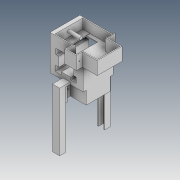
# Autodesk Inventor part: Peça16
Saved by Autodesk Inventor 2021 (Build 250183000, 183)
## iProperties
Created: 2020-10-08
Part Number: Peça16
Material: Genérico
Document SubType Name: Modeling
Designer: evert
Density: 1 g/cm^3
Appearance: Padrão
Author: evert
Autodesk Inventor part; units mm, degrees
ref_plane "YZ Plane" through (0, 0, 0) normal (1, 0, 0) x (0, 1, 0)
ref_plane "XZ Plane" through (0, 0, 0) normal (0, 1, 0) x (-1, 0, 0)
ref_plane "XY Plane" through (0, 0, 0) normal (0, 0, 1) x (1, 0, 0)
sketch "Esboço2" plane through (0, 0, 0) normal (0, 0, 1) x (1, 0, 0)
  line L0 (0, 0) -> (-5, 0)
  line L1 (-5, 0) -> (-5, -5)
  line L2 (-5, -5) -> (-2, -5)
  line L3 (-2, -5) -> (-2, -15)
  line L4 (-2, -15) -> (-5.6275, -15)
  line L5 (-5.6275, -15) -> (-5.6275, -20)
  line L6 (-5.6275, -20) -> (0, -20)
  line L7 (0, -20) -> (0, -17.5)
  line L8 (0, -17.5) -> (10, -17.5)
  line L9 (10, -17.5) -> (10, -20)
  line L10 (10, -20) -> (15, -20)
  line L11 (15, -20) -> (15, -15)
  line L12 (15, -15) -> (12.5, -15)
  line L13 (12.5, -15) -> (12.5, -5)
  line L14 (12.5, -5) -> (15, -5)
  line L15 (15, 0) -> (15, -5)
  line L16 (15, 0) -> (10, 0)
  line L17 (10, 0) -> (10, -2.5)
  line L18 (10, -2.5) -> (0, -2.5)
  line L19 (0, -2.5) -> (0, 0)
  line L20 (-2.2, -14.8) -> (-2.2, -5.2)
  line L21 (-2.2, -5.2) -> (-4.7, -5.2)
  line L22 (-2.2, -14.8) -> (-4.7, -14.8)
  line L23 (-2.2, -14.8) -> (-5.8275, -14.8)
  line L24 (-5.8275, -14.8) -> (-5.8275, -20)
  line L25 (-5.8275, -20) -> (-5.8275, -20.2)
  line L26 (-5.8275, -20.2) -> (0.2, -20.2)
  line L27 (0.2, -20.2) -> (0.2, -17.7)
  line L28 (0.2, -17.7) -> (9.8, -17.7)
  line L29 (9.8, -17.7) -> (9.8, -18.4636)
  line L30 (9.8, -18.4636) -> (9.8, -20.2)
  line L31 (9.8, -20.2) -> (15.2, -20.2)
  line L32 (15.2, -20.2) -> (15.2, -14.8)
  line L33 (15.2, -14.8) -> (12.7, -14.8)
  line L34 (12.7, -14.8) -> (12.7, -5.2)
  line L35 (12.7, -5.2) -> (15.1265, -5.2)
  line L36 (15.1265, -5.2) -> (15.2, -5.2)
  line L37 (15.2, -5.2) -> (15.2, 0)
  line L38 (-4.7, -5.2) -> (-5.2, -5.2)
  line L39 (-5.2, -5.2) -> (-5.2, 0)
  line L40 (-12.2, 0) -> (-12.2, -24.2)
  line L41 (-12.2, -24.2) -> (22.2, -24.2)
  line L42 (22.2, -24.2) -> (22.2, 0)
  line L43 (15.2, 0) -> (15.2, 0.2)
  line L44 (15.2, 0.2) -> (13.2, 0.2)
  line L45 (22.2, 0) -> (22.2, 1)
  line L46 (22.2, 1) -> (13.2, 1)
  line L47 (13.2, 1) -> (13.2, 0.2)
  line L48 (-12.2, 0) -> (-12.2, 1.2)
  line L49 (-5.2, 0) -> (-5.2, 0.2)
  line L50 (-5.2, 0.2) -> (-3.2, 0.2)
  line L51 (-3.2, 1.2) -> (-12.2, 1.2)
  line L52 (-3.2, 1.2) -> (0, 1.2)
  line L53 (0, 1.2) -> (0, 0.2)
  line L54 (0, 0.2) -> (-3.2, 0.2)
  line L55 (0.5946, -2.5) -> (0.5946, 9.5)
  line L56 (0.5946, 9.5) -> (9.5946, 9.5)
  line L57 (9.5946, 9.5) -> (9.5946, -2.5)
  line L58 (0.5946, -2.5) -> (9.5946, -2.5)
  dimension "d0" = 5
  dimension "d1" = 5
  dimension "d2" = 3
  dimension "d3" = 10
  dimension "d4" = 5
  dimension "d5" = 2.5
  dimension "d6" = 10
  dimension "d7" = 5
  dimension "d8" = 5
  dimension "d9" = 10
  dimension "d11" = 5
  dimension "d12" = 0.2
  dimension "d13" = 0.2
  dimension "d14" = 0.2
  dimension "d15" = 0.2
  dimension "d16" = 0.2
  dimension "d17" = 0.2
  dimension "d19" = 0.2
  dimension "d20" = 0.2
  dimension "d21" = 0.2
  dimension "d22" = 0.2
  dimension "d23" = 0.2
  dimension "d24" = 0.2
  dimension "d25" = 0.2
  dimension "d26" = 0.2
  dimension "d27" = 0.2
  dimension "d28" = 7
  dimension "d29" = 4
  dimension "d30" = 7
  dimension "d31" = 0.2
  dimension "d32" = 2
  dimension "d33" = 1
  dimension "d34" = 0.2
  dimension "d35" = 2
  dimension "d36" = 1
  dimension "d39" = 12
  dimension "d40" = 9
  constraints: 118 end point, 27 perpendicular, 16 point on line, 9 horizontal, 8 vertical, 3 parallel, 1 collinear
  measures "d0" distance of L0.start L0.end
  measures "d1" distance of L0.end L1.end
  measures "d2" distance of L1.end L2.end
  measures "d3" distance of L2.end L3.end
  measures "d4" distance of L4.end L5.end
  measures "d5" distance of L6.end L7.end
  measures "d6" distance of L7.end L8.end
  measures "d7" distance of L9.end L10.end
  measures "d8" distance of L10.end L11.end
  measures "d9" distance of L12.end L13.end
  measures "d11" distance of L15.start L16.end
  measures "d12" distance between parallel lines of L3 L20
  measures "d13" distance between parallel lines of L21 L2
  measures "d14" distance between parallel lines of L4 L22
  measures "d15" distance between parallel lines of L5 L24
  measures "d16" distance between parallel lines of L6 L26
  measures "d17" distance between parallel lines of L7 L27
  measures "d19" distance between parallel lines of L8 L28
  measures "d20" distance between parallel lines of L9 L29
  measures "d21" distance between parallel lines of L31 L10
  measures "d22" distance between parallel lines of L11 L32
  measures "d23" distance between parallel lines of L12 L33
  measures "d24" distance between parallel lines of L34 L13
  measures "d25" distance between parallel lines of L35 L14
  measures "d26" distance between parallel lines of L37 L15
  measures "d27" distance between parallel lines of L1 L39
  measures "d28" distance of L39.end L40.start
  measures "d29" distance from line of L41 L25.end
  measures "d30" distance from line of L42 L31.end
  measures "d31" distance of L37.end L43.end
  measures "d32" distance of L43.end L44.end
  measures "d33" distance of L42.end L45.end
  measures "d34" distance of L39.end L49.end
  measures "d35" distance of L49.end L50.end
  measures "d36" distance between parallel lines of L50 L51
  measures "d39" distance of L55.start L55.end
  measures "d40" distance of L55.end L56.end
extrude "Extrusão1" add sketch "Esboço2" along normal blind 30 contours L22 L23 L24 L25 L26 L27 L28 L29 L30 L31 L32 L33 L34 L35 L36 L37 L43 L44 L47 L46 L45 L42 L41 L40 L48 L51 L52 L53 L54 L50 L49 L39 L38 L21 L20
sketch "Esboço4" plane through (-12.2, -24.2, 0) normal (-1, 0, 0) x (0, 0, 1)
  circle A0 centre (30, 27.7) radius 6 projected
  line L0 (30, 27.7) -> (0, 27.7)
  line L1 (15, 27.7) -> (15, 25.4)
  line L2 (0, 25.4) -> (30, 25.4) projected
  line L3 (0, 27.7) -> (30, 27.7)
  line L4 (30, 27.7) -> (30, 25.4)
  line L5 (30, 25.4) -> (0, 25.4)
  line L6 (0, 25.4) -> (0, 27.7)
  point P0 (0, 24.2)
  constraints: 12 end point, 2 horizontal, 2 midpoint, 2 parallel, 1 perpendicular
extrude "Extrusão2" add sketch "Esboço4" against normal blind 5 contours L0 L4 L2 A0 | A0 L2 L1 L0 | L1 L2 L6 L0 picked at (28.1528, 26.1667)
sketch "Esboço5" plane through (-7.2, -24.2, 0) normal (1, 0, 0) x (0, 0, -1)
  line L0 (-30, 27.7) -> (0, 27.7) projected
  line L1 (0, 27.7) -> (-15, 27.7)
  circle A0 centre (-15, 27.7) radius 1.5
  point P0 (0, 24.2)
  dimension "d48" = 3
  constraints: 2 end point, 1 centre point, 1 coincident, 1 midpoint
  measures "d48" diameter of A0
extrude "Extrusão3" add sketch "Esboço5" along normal blind 12.2
sketch "Esboço6" plane through (-7.2, -24.2, 0) normal (-1, 0, 0) x (0, 0, 1)
  line L0 (13.5, 27.7) -> (16.5, 27.7) projected
  circle A0 centre (15, 27.7) radius 1.5
  point P0 (0, 24.2)
  constraints: 1 centre point, 1 midpoint
extrude "Extrusão4" add sketch "Esboço6" along normal blind 5 contours A0 L0 picked at (15.4855, 27.8197)
sketch "Esboço7" plane through (-12.2, -24.2, 0) normal (-1, 0, 0) x (0, 0, 1)
  circle A0 centre (30, 27.7) radius 6 projected
  line L0 (13.5, 27.7) -> (0, 27.7) projected
  line L1 (30, 33.7) -> (0, 33.7)
  line L2 (0, 33.7) -> (0, 27.7)
  line L3 (0, 27.7) -> (30, 27.7)
  line L4 (30, 27.7) -> (30, 33.7)
  point P0 (0, 24.2)
  constraints: 8 end point, 2 parallel, 1 horizontal, 1 perpendicular, 1 vertical alignment, 1 other
extrude "Extrusão5" add sketch "Esboço7" against normal blind 5 contours L4 L3 A0 | A0 L3 L0 L2 L1 picked at (26.0501, 28.145)
sketch "Esboço8" plane through (-12.2, -24.2, 0) normal (-1, 0, 0) x (0, 0, 1)
  line L0 (30, 33.7) -> (0, 33.7) projected
  line L1 (0, 33.7) -> (0, 35.2)
  line L2 (0, 35.2) -> (30, 35.2)
  line L3 (30, 35.2) -> (30, 33.7)
  line L4 (30, 33.7) -> (0, 33.7)
  line L5 (30, 33.7) -> (30, 25.4) projected
  point P0 (0, 24.2)
  dimension "d55" = 1.5
  constraints: 8 end point, 3 perpendicular, 1 vertical
  measures "d55" distance of L0.end L1.end
extrude "Extrusão6" add sketch "Esboço8" against normal blind 5
sketch "Esboço10" plane through (13.2, 1, 0) normal (0, 1, 0) x (1, 0, 0)
  line L0 (-8.2, -16.5) -> (-8.2, -13.5) projected
  line L1 (-8.2, -15) -> (-8.2, -21.5)
  line L2 (-8.2, -15) -> (-8.2, -8.5)
  line L3 (0, 0) -> (0, -30) projected
  line L4 (0, 0) -> (-13.2, 0)
  line L5 (-3.4, 0) -> (-13, 0) projected
  line L6 (-13.2, 0) -> (-13.2, -8.5)
  line L7 (-13, 0) -> (-13, -30) projected
  line L8 (-13.2, -8.5) -> (0, -8.5)
  line L9 (0, -8.5) -> (0, 0)
  line L10 (2, -30) -> (-3.4, -30) projected
  line L11 (0, -30) -> (0, -21.5)
  line L12 (0, -21.5) -> (-13.2, -21.5)
  line L13 (-13.2, 0) -> (-13.2, -30) projected
  line L14 (-13.2, -21.5) -> (-13.2, -30)
  line L15 (-13.2, -30) -> (0, -30)
  dimension "d58" = 6.5
  dimension "d59" = 6.5
  constraints: 20 end point, 5 perpendicular, 5 point on line, 2 collinear, 1 midpoint, 1 parallel
  measures "d58" distance of L1.start L1.end
  measures "d59" distance of L1.start L2.end
extrude "Extrusão7" add sketch "Esboço10" against normal blind 0.8 contours L12 L3 L10 L15 L7 | L7 L15 L13 L12 | L8 L7 L4 L3 | L8 L6 L4 L7
sketch "Esboço15" plane through (22.2, -24.2, 0) normal (1, 0, 0) x (0, 0, -1)
  line L0 (-30, 25.2) -> (-21.5, 25.2) projected
  line L1 (-30, 25.2) -> (0, 25.2)
  line L2 (0, 25.2) -> (0, 24.2)
  line L3 (0, 24.2) -> (-30, 24.2)
  line L4 (-30, 24.2) -> (-30, 25.2)
  constraints: 8 end point, 2 parallel, 1 horizontal, 1 perpendicular
extrude "Extrusão10" add sketch "Esboço15" along normal blind 3
sketch "Esboço16" plane through (0, 1, 8.5) normal (0, 1, 0) x (1, 0, 0)
  line L0 (22.2, -21.5) -> (25.2, -21.5) projected
  line L1 (25.2, 8.5) -> (23.7, 8.5)
  line L2 (23.7, -21.5) -> (25.2, -21.5)
  line L3 (0, -21.5) -> (25.2, -21.5) projected
  line L4 (-12.2, -21.5) -> (-12.2, 8.5) projected
  line L5 (25.2, -21.5) -> (-12.2, -21.5)
  line L6 (-12.2, -21.5) -> (-12.2, -20.5)
  line L7 (-12.2, -20.5) -> (25.2, -20.5)
  line L8 (25.2, -20.5) -> (25.2, -21.5)
  line L9 (0, 8.5) -> (25.2, 8.5) projected
  line L10 (25.2, 8.5) -> (-12.2, 8.5)
  line L11 (-12.2, 8.5) -> (-12.2, 7.5)
  line L12 (-12.2, 7.5) -> (25.2, 7.5)
  line L13 (25.2, 7.5) -> (25.2, 8.5)
  line L14 (25.2, 8.5) -> (24.2, 8.5)
  line L15 (24.2, 8.5) -> (24.2, -21.5)
  line L16 (24.2, -21.5) -> (25.2, -21.5)
  line L17 (25.2, -21.5) -> (25.2, 8.5)
  point P0 (24.2, 7.5)
  point P1 (24.2, -20.5)
  dimension "d70" = 1
  dimension "d71" = 1
  dimension "d73" = 1
  constraints: 28 end point, 7 parallel, 4 horizontal, 3 perpendicular, 3 point on line, 1 midpoint
  measures "d70" distance between parallel lines of L9 L12
  measures "d71" distance between parallel lines of L7 L3
  measures "d73" distance of L16.end L15.end
extrude "Extrusão11" add sketch "Esboço16" along normal blind 10 contours L3 L5 L4 L7 L15 L0 | L15 L7 L8 L0 | L15 L12 L17 L7 | L15 L1 L13 L12 | L12 L4 L10 L9 L1 L15
sketch "Esboço18" plane through (0, 0, 30) normal (0, 0, 1) x (1, 0, 0)
  line L0 (-12.2, 11) -> (-12.2, -24.2) projected
  line L1 (-12.2, -24.2) -> (22.2, -24.2) projected
  line L2 (-12.2, 11) -> (-11.2, 11)
  line L3 (-11.2, 11) -> (-11.2, -24.2)
  line L4 (-11.2, -24.2) -> (-12.2, -24.2)
  line L5 (-12.2, -24.2) -> (-12.2, 11)
  point P0 (0, 0)
  dimension "d76" = 1
  constraints: 8 end point, 2 parallel, 1 horizontal, 1 perpendicular, 1 point on line
  measures "d76" distance of L3.end L4.end
extrude "Extrusão12" cut sketch "Esboço18" against normal through all
sketch "Esboço20" plane through (0, 1, 8.5) normal (0, 1, 0) x (1, 0, 0)
  line L0 (0, 7.5) -> (0, -20.5) projected
  line L1 (12.7, 8.5) -> (12.7, -21.5) projected
  line L2 (0, 0) -> (12.7, 0)
  line L3 (12.7, 0) -> (12.7, 1)
  line L4 (12.7, 1) -> (0, 1)
  line L5 (0, 1) -> (0, 0)
  line L6 (0, 0) -> (13.2, 0) projected
  line L7 (12.7, 1) -> (13.2, 1)
  line L8 (13.2, 1) -> (13.2, 0)
  line L9 (13.2, 0) -> (12.7, 0)
  line L10 (12.7, 0) -> (12.7, 1)
  line L11 (13.2, 0) -> (13.2, -13) projected
  line L12 (0, -20.5) -> (0, -13) projected
  line L13 (13.2, -13) -> (0, -13)
  line L14 (0, -13) -> (0, -14)
  line L15 (0, -14) -> (13.2, -14)
  line L16 (13.2, -14) -> (13.2, -13)
  point P0 (0, 8.5)
  point P1 (0, -14)
  point P2 (0, -13)
  point P3 (0, 1)
  dimension "d79" = 1
  dimension "d80" = 1
  constraints: 24 end point, 6 parallel, 3 horizontal, 3 perpendicular, 3 point on line
  measures "d79" distance between parallel lines of L4 L2
  measures "d80" distance between parallel lines of L15 L13
extrude "Extrusão13" cut sketch "Esboço20" against normal blind 1 contours L4 L1 L2 L0 | L7 L8 L6 L1 | L13 L1 L15 L0 | L13 L16 L15 L1
sketch "Esboço38" plane through (22.2, -24.2, 0) normal (0, -1, 0) x (1, 0, 0)
  line L0 (-33.4, 0) -> (-33.4, 30) projected
  line L1 (0, 0) -> (-33.4, 0)
  line L2 (-33.4, 0) -> (-33.4, 30)
  line L3 (-33.4, 30) -> (0, 30)
  line L4 (0, 30) -> (0, 0)
  line L5 (0, 0) -> (0, 3.5)
  line L6 (-33.4, 30) -> (0, 30) projected
  line L7 (0, 30) -> (0, 26.5)
  line L8 (0, 26.5) -> (0, 3.5)
  line L9 (0, 3.5) -> (-16.5, 3.5)
  line L10 (0, 26.5) -> (-16.5, 26.5)
  line L11 (-16.5, 3.5) -> (-16.5, 26.5)
  line L12 (0, 3.5) -> (0, 3)
  line L13 (0, 0) -> (0, 30) projected
  line L14 (0, 3) -> (-17, 3)
  line L15 (-17, 3) -> (-17, 3.5)
  line L16 (-17, 3.5) -> (-16.5, 3.5)
  line L17 (0, 26.5) -> (0, 27)
  line L18 (0, 27) -> (-17, 27)
  line L19 (-17, 27) -> (-17, 26.5)
  line L20 (-17, 26.5) -> (-16.5, 26.5)
  line L21 (0, 3.5) -> (-0.5, 3.5)
  line L22 (-0.5, 3.5) -> (-0.5, 26.5)
  point P0 (-22.2, 0)
  point P1 (0, 27)
  dimension "d128" = 3.5
  dimension "d129" = 3.5
  dimension "d131" = 16.5
  dimension "d132" = 16.5
  dimension "d133" = 0.5
  dimension "d134" = 17
  dimension "d135" = 0.5
  constraints: 40 end point, 8 point on line, 6 perpendicular, 3 horizontal, 2 parallel, 1 vertical
  measures "d128" distance of L1.start L5.end
  measures "d129" distance of L6.end L7.end
  measures "d131" distance of L5.end L9.end
  measures "d132" distance of L7.end L10.end
  measures "d133" distance of L5.end L12.end
  measures "d134" distance of L12.end L14.end
  measures "d135" distance of L7.end L17.end
extrude "Extrusão25" add sketch "Esboço38" along normal blind 12 contours L14 L15 L16 L9 L4 | L4 L10 L20 L19 L18 | L9 L22 L10 L4
sketch "Esboço39" plane through (22.2, -36.2, 0) normal (0, -1, 0) x (1, 0, 0)
  line L0 (-17, 3) -> (0, 3) projected
  line L1 (0, 27) -> (-17, 27) projected
  line L2 (0, 3) -> (-17, 3)
  line L3 (-17, 3) -> (-17, 27)
  line L4 (-17, 27) -> (0, 27)
  line L5 (0, 27) -> (0, 3)
  point P0 (-22.2, 0)
  point P1 (-17, 3)
  constraints: 8 end point, 2 parallel, 1 horizontal, 1 perpendicular
extrude "Extrusão26" add sketch "Esboço39" along normal blind 1
sketch "Esboço40" plane through (5.2, -24.2, 27) normal (0, 0, 1) x (1, 0, 0)
  line L0 (0, -13) -> (17, -13) projected
  line L1 (0, 0) -> (16.5, 0) projected
  line L2 (0, -13) -> (1, -13)
  line L3 (1, -13) -> (1, 0)
  line L4 (1, 0) -> (0, 0)
  line L5 (0, 0) -> (0, -13)
  point P0 (-5.2, 24.2)
  point P1 (1, -13)
  dimension "d140" = 1
  constraints: 8 end point, 2 parallel, 1 horizontal, 1 perpendicular, 1 point on line
  measures "d140" distance of L4.end L3.end
extrude "Extrusão27" add sketch "Esboço40" along normal blind 5
sketch "Esboço41" plane through (22.2, -24.2, 3) normal (0, 0, -1) x (-1, 0, 0)
  line L0 (17, 0) -> (17, -13) projected
  line L1 (16, 0) -> (16, -13) projected
  line L2 (17, 0) -> (16, 0)
  line L3 (16, 0) -> (16, -13)
  line L4 (16, -13) -> (17, -13)
  line L5 (17, -13) -> (17, 0)
  point P0 (22.2, 24.2)
  constraints: 8 end point, 2 parallel, 1 horizontal, 1 perpendicular
extrude "Extrusão28" add sketch "Esboço41" along normal blind 5
sketch "Esboço42" plane through (5.2, -36.2, 3.5) normal (-1, 0, 0) x (0, 0, 1)
  line L0 (-5.5, -1) -> (-5.5, 12) projected
  line L1 (-5.5, 12) -> (-5.5, 6.1)
  line L2 (-5.5, 6.1) -> (0, 6.1)
  line L3 (0, 12) -> (0, 0) projected
  line L4 (0, 6.1) -> (28.5, 6.1)
  line L5 (28.5, -1) -> (28.5, 12) projected
  line L6 (-5.5, 6.1) -> (-2.75, 6.1)
  circle A0 centre (-2.75, 6.1) radius 0.5
  line L7 (28.5, 6.1) -> (25.75, 6.1)
  circle A1 centre (25.75, 6.1) radius 0.5
  point P0 (-3.5, 36.2)
  dimension "d145" = 5.9
  dimension "d146" = 1
  dimension "d147" = 2.75
  dimension "d148" = 1
  constraints: 10 end point, 5 point on line, 2 centre point, 2 coincident, 1 horizontal, 1 midpoint
  measures "d145" distance of L0.end L1.end
  measures "d146" diameter of A0
  measures "d147" distance of L4.end L7.end
  measures "d148" diameter of A1
extrude "Extrusão29" cut sketch "Esboço42" against normal blind 5
sketch "Esboço46" plane through (22.2, -37.2, 0) normal (0, -1, 0) x (1, 0, 0)
  line L0 (-17, -2) -> (-17, 32) projected
  line L1 (-17, 26.9875) -> (-19, 26.9875)
  line L2 (-22.2, 29) -> (-22.2, 22.5) projected
  line L3 (-19, 26.9875) -> (-19, 3.5)
  line L4 (-17, 0) -> (-17, 3.5) projected
  line L5 (-19, 3.5) -> (-17, 3.5)
  point P0 (-22.2, 0)
  dimension "d152" = 2
  constraints: 6 end point, 3 perpendicular, 1 point on line
  measures "d152" distance of L1.start L1.end
extrude "Extrusão30" add sketch "Esboço46" against normal blind 1
sketch "Esboço47" plane through (22.2, -37.2, 0) normal (0, -1, 0) x (1, 0, 0)
  line L0 (-16.7452, 15.2437) -> (-16.7452, 11.1125)
  line L1 (-16.7452, 11.1125) -> (-16.7452, 15.2437)
  line L2 (-16.7452, 19.05) -> (-16.7452, 15.2437)
  line L3 (-16.7452, 15.2437) -> (-16.7452, 17.2437)
  line L4 (-16.7452, 17.2437) -> (-17.2452, 17.2437)
  line L5 (-17.2452, 17.2437) -> (-16.7452, 17.2437)
  line L6 (-16.7452, 17.2437) -> (-16.2452, 17.2437)
  line L7 (-16.2452, 17.2437) -> (-16.2452, 16.2437)
  line L8 (-29.4, 16.5) -> (-17.2, 16.5) projected
  line L9 (-16.2452, 16.2437) -> (-17.2452, 16.2437)
  line L10 (-17.2452, 16.2437) -> (-17.2452, 17.2437)
  line L11 (-16.7452, 15.2437) -> (-16.7452, 13.2437)
  line L12 (-16.7452, 13.2437) -> (-17.2452, 13.2437)
  line L13 (-17.2452, 13.2437) -> (-16.7452, 13.2437)
  line L14 (-16.2452, 13.2437) -> (-16.7452, 13.2437)
  line L15 (-29.4, 13.5) -> (-17.2, 13.5) projected
  line L16 (-16.2452, 13.2437) -> (-16.2452, 14.2437)
  line L17 (-16.2452, 14.2437) -> (-17.2452, 14.2437)
  line L18 (-17.2452, 14.2437) -> (-17.2452, 13.2437)
  point P0 (-22.2, 0)
  dimension "d155" = 2
  dimension "d156" = 0.5
  dimension "d157" = 0.5
  dimension "d158" = 2
  constraints: 34 end point, 9 point on line, 7 perpendicular, 4 collinear, 1 parallel, 1 vertical
  measures "d155" distance of L0.start L3.end
  measures "d156" distance of L3.end L4.end
  measures "d157" distance of L3.end L6.end
  measures "d158" distance of L0.start L11.end
extrude "Extrusão31" add sketch "Esboço47" along normal blind 3
sketch "Esboço48" plane through (5.9548, -37.2, 16.2437) normal (0, 0, -1) x (-1, 0, 0)
  line L0 (0, -3) -> (1, -3) projected
  circle A0 centre (0.5, -3) radius 0.5
  point P0 (5.9548, 37.2)
  dimension "d161" = 1
  constraints: 1 centre point, 1 midpoint
  measures "d161" diameter of A0
extrude "Extrusão32" add sketch "Esboço48" along normal blind 3 and the other way blind 1
sketch "Esboço53" plane through (0, 1, 29) normal (0, 1, 0) x (1, 0, 0)
  line L0 (13.2, 21.5) -> (13.2, 6.5) projected
  line L1 (13.2, 21.5) -> (11.2, 21.5)
  line L2 (13.2, 21.5) -> (0, 21.5) projected
  line L3 (11.2, 21.5) -> (11.2, 6.5)
  line L4 (0, 6.5) -> (13.2, 6.5) projected
  line L5 (13.2, 6.5) -> (11.2, 6.5)
  line L6 (13.2, 6.5) -> (13.2, 21.5)
  point P0 (0, 29)
  dimension "d169" = 2
  constraints: 8 end point, 3 perpendicular, 2 point on line
  measures "d169" distance of L0.start L1.end
extrude "Extrusão34" add sketch "Esboço53" against normal blind 0.8
sketch "Esboço54" plane through (25.2, 11, 30) normal (0, 1, 0) x (1, 0, 0)
  line L0 (-1, 1) -> (-1, 29) projected
  line L1 (-1, 1) -> (0, 1)
  line L2 (0, 1) -> (0, 29)
  line L3 (0, 0) -> (0, 30) projected
  line L4 (-1, 29) -> (-25.2, 29) projected
  line L5 (-1, 29) -> (0, 29)
  line L6 (-25.2, 1) -> (-1, 1) projected
  line L7 (-1, 29) -> (-1, 1)
  point P0 (-25.2, 30)
  constraints: 8 end point, 1 collinear, 1 horizontal, 1 perpendicular, 1 point on line
extrude "Extrusão35" cut sketch "Esboço54" against normal blind 10
sketch "Esboço57" plane through (-7.2, -24.2, 0) normal (1, 0, 0) x (0, 0, -1)
  line L0 (-1, 25.4) -> (-1, 35.2) projected
  circle A0 centre (-15, 27.7) radius 1.5 projected
  circle A1 centre (-15, 30.7) radius 1.5
  line L1 (-15, 27.7) -> (-15, 30.7)
  point P0 (0, 24.2)
  dimension "d175" = 3
  constraints: 2 end point, 1 centre point, 1 vertical
  measures "d175" diameter of A1
extrude "Extrusão36" add sketch "Esboço57" along normal blind 12.2 contours A1
sketch "Esboço58" plane through (5, 3.5, 15) normal (1, 0, 0) x (0, 0, -1)
  circle A0 centre (0, 0) radius 1.5 projected
  circle A1 centre (0, 0) radius 1.5
  point P0 (15, -3.5)
  point P1 (0, 1.5)
  constraints: 1 centre point, 1 coincident, 1 vertical alignment
extrude "Extrusão37" cut sketch "Esboço58" against normal blind 12.2
sketch "Esboço59" plane through (0, 1, 29) normal (0, 1, 0) x (1, 0, 0)
  line L0 (0, 21.5) -> (11.2, 21.5) projected
  line L1 (0, 21.5) -> (11.2, 21.5)
  line L2 (11.2, 21.5) -> (11.2, 24.5)
  line L3 (11.2, 24.5) -> (0, 24.5)
  line L4 (0, 24.5) -> (0, 21.5)
  line L5 (11.2, 6.5) -> (11.2, 21.5) projected
  line L6 (0, 0) -> (0, 6.5) projected
  line L7 (11.2, 6.5) -> (0, 6.5)
  line L8 (0, 6.5) -> (0, 3.25)
  line L9 (11.2, 6.5) -> (11.2, 3.5)
  line L10 (11.2, 3.5) -> (0, 3.5)
  point P0 (0, 29)
  point P1 (11.2, 21.5)
  point P2 (0, 3.5)
  dimension "d180" = 3
  dimension "d181" = 3
  constraints: 16 end point, 3 perpendicular, 2 horizontal, 2 parallel, 1 midpoint, 1 point on line, 1 vertical
  measures "d180" distance of L1.end L2.end
  measures "d181" distance of L5.start L9.end
extrude "Extrusão38" cut sketch "Esboço59" against normal blind 1
sketch "Esboço60" plane through (0, 1, 29) normal (0, 1, 0) x (1, 0, 0)
  line L0 (25.2, -1) -> (25.2, 29) projected
  line L1 (25.2, 29) -> (25.2, 19.54)
  line L2 (25.2, 19.54) -> (36.7, 19.54)
  line L3 (36.7, 19.54) -> (36.7, 0)
  line L4 (36.7, 0) -> (25.4, 0)
  line L5 (25.4, 0) -> (36.7, 0)
  line L6 (36.7, 19.54) -> (36.7, -2.46)
  line L7 (36.7, -2.46) -> (25.2, -2.46)
  line L8 (25.2, -2.46) -> (25.2, 19.54)
  point P0 (0, 29)
  dimension "d184" = 9.46
  dimension "d185" = 11.5
  dimension "d186" = 22
  dimension "d187" = 11.5
  constraints: 16 end point, 2 point on line, 1 horizontal, 1 parallel, 1 perpendicular, 1 vertical
  measures "d184" distance of L0.end L1.end
  measures "d185" distance of L1.end L2.end
  measures "d186" distance of L2.end L6.end
  measures "d187" distance of L6.end L7.end
extrude "Extrusão39" add sketch "Esboço60" against normal blind 1
sketch "Esboço62" plane through (-7.2, 11, 29) normal (0, 1, 0) x (1, 0, 0)
  line L0 (19.9, 29) -> (19.9, -1) projected
  line L1 (19.9, -1) -> (19.9, -4.091)
  line L2 (22.4, -1) -> (19.9, -1) projected
  line L3 (19.9, 0) -> (19.9, -1)
  line L4 (-4, -1) -> (32.4, -1) projected
  line L5 (19.9, -1) -> (32.4, -1)
  line L6 (7.2, 0) -> (32.4, 0) projected
  line L7 (32.4, -1) -> (32.4, 0)
  line L8 (32.4, 0) -> (19.9, 0)
  line L9 (32.4, 28) -> (32.4, 0) projected
  line L10 (32.4, 28) -> (32.4, 29)
  line L11 (29.4, 29) -> (32.4, 29) projected
  line L12 (32.4, 29) -> (29.4, 29)
  line L13 (29.4, 29) -> (29.4, 28)
  line L14 (32.4, 28) -> (7.2, 28) projected
  point P0 (7.2, 29)
  point P1 (32.4, 20.04)
  constraints: 16 end point, 3 collinear, 2 perpendicular, 2 point on line, 2 vertical
extrude "Extrusão41" cut sketch "Esboço62" against normal blind 10 contours L6 L7 L4 L2 L0 | L13 L11 L10 L14
sketch "Esboço64" plane through (0, 1, 4.5) normal (0, 1, 0) x (1, 0, 0)
  line L0 (22.3, -4.46) -> (25.2, -4.46) projected
  line L1 (22.2, 4.5) -> (25.2, 4.5) projected
  line L2 (22.3, -4.46) -> (25.2, -4.46)
  line L3 (25.2, -4.46) -> (25.2, 4.5)
  line L4 (25.2, 4.5) -> (22.3, 4.5)
  line L5 (22.3, 4.5) -> (22.3, -4.46)
  point P0 (0, 4.5)
  constraints: 8 end point, 2 parallel, 1 horizontal, 1 perpendicular
extrude "Extrusão43" cut sketch "Esboço64" against normal blind 12
sketch "Esboço65" plane through (0, 1, 4.5) normal (0, 1, 0) x (1, 0, 0)
  line L0 (37.2, -4.46) -> (37.2, -27.46)
  line L1 (25.2, -27.46) -> (37.2, -27.46) projected
  line L2 (37.2, -27.46) -> (22.3, -27.46)
  line L3 (22.3, -31.96) -> (22.3, -27.46) projected
  line L4 (22.3, -27.46) -> (22.3, -31.96)
  line L5 (12.7, -25.5) -> (12.7, -24.5) projected
  line L6 (12.7, -31.96) -> (12.7, -25.5)
  line L7 (12.7, -25.5) -> (25.2, -25.5)
  line L8 (15.2, 4.5) -> (15.2, -25.5) projected
  line L9 (25.2, -26.96) -> (25.2, -25.5) projected
  line L10 (25.2, -25.5) -> (25.2, -26.96)
  line L11 (36.7, -26.96) -> (25.2, -26.96) projected
  line L12 (25.2, -26.96) -> (36.7, -26.96)
  line L13 (36.7, -4.96) -> (36.7, -26.96) projected
  line L14 (36.7, -26.96) -> (36.7, -4.96)
  line L15 (36.7, -4.96) -> (21.8, -4.96)
  line L16 (25.2, -4.96) -> (36.7, -4.96) projected
  line L17 (21.8, -4.96) -> (21.8, 0.04) projected
  line L18 (21.8, -4.96) -> (21.8, 0.04)
  line L19 (21.8, 0.04) -> (22.3, 0.04)
  line L20 (22.3, 4.5) -> (22.3, -4.46) projected
  line L21 (22.3, 0.04) -> (22.3, -4.46)
  line L22 (22.3, -4.46) -> (37.2, -4.46)
  line L23 (12.7, 4.5) -> (12.7, -25.5) projected
  line L24 (12.7, -25.5) -> (12.7, -31.96)
  line L25 (12.7, -31.96) -> (12.7, -32.46)
  line L26 (12.7, -32.46) -> (22.3, -32.46)
  line L27 (22.3, -32.46) -> (22.3, -31.96)
  point P0 (0, 4.5)
  dimension "d210" = 0.5
  constraints: 34 end point, 7 collinear, 7 perpendicular, 2 point on line
  measures "d210" distance of L6.start L25.end
extrude "Extrusão44" add sketch "Esboço65" against normal blind 1
sketch "Esboço67" plane through (0, 1, 4.5) normal (0, 1, 0) x (1, 0, 0)
  line L0 (22.2, 3.5) -> (0, 3.5) projected
  line L1 (21.8, 3.5) -> (22.3, 3.5)
  line L2 (22.3, 4.5) -> (22.3, -4.46) projected
  line L3 (22.2, 4.5) -> (22.3, 4.5) projected
  line L4 (22.3, 4.5) -> (24.3, 4.5)
  line L5 (24.3, 4.5) -> (24.3, -2.46)
  line L6 (24.3, -2.46) -> (39.2, -2.46)
  line L7 (37.2, -4.46) -> (22.3, -4.46) projected
  line L8 (39.2, -2.46) -> (39.2, -29.46)
  line L9 (39.2, -29.46) -> (23.2371, -29.46)
  line L10 (23.2371, -29.46) -> (23.2371, -34.46)
  line L11 (23.2371, -34.46) -> (12.7, -34.46)
  line L12 (12.7, -32.46) -> (12.7, -25.5) projected
  line L13 (12.7, -34.46) -> (12.7, -32.46)
  line L14 (25.2, -27.46) -> (37.2, -27.46) projected
  line L15 (37.2, -27.46) -> (37.2, -4.46) projected
  line L16 (12.7, -32.46) -> (22.3, -32.46) projected
  line L17 (22.3, 4.5) -> (22.3, -4.46)
  line L18 (22.3, -4.46) -> (37.2, -4.46) projected
  line L19 (22.3, -4.46) -> (37.2, -4.46)
  line L20 (37.2, -4.46) -> (37.2, -27.46) projected
  line L21 (37.2, -4.46) -> (37.2, -27.46)
  line L22 (22.3, -31.96) -> (22.3, -27.46) projected
  line L23 (37.2, -27.46) -> (22.3, -27.46)
  line L24 (22.3, -32.46) -> (22.3, -27.46)
  line L25 (22.3, -32.46) -> (12.7, -32.46)
  point P0 (0, 4.5)
  dimension "d218" = 2
  dimension "d219" = 2
  dimension "d220" = 2
  dimension "d221" = 2
  dimension "d222" = 2
  constraints: 30 end point, 7 perpendicular, 3 collinear, 3 horizontal, 1 point on line, 1 vertical
  measures "d218" distance of L2.start L4.end
  measures "d219" distance between parallel lines of L6 L7
  measures "d220" distance between parallel lines of L14 L9
  measures "d221" distance between parallel lines of L8 L15
  measures "d222" distance between parallel lines of L11 L16
extrude "Extrusão46" add sketch "Esboço67" against normal blind 1
sketch "Esboço68" plane through (0, 1, 4.5) normal (0, 1, 0) x (1, 0, 0)
  line L0 (24.3, 4.5) -> (22.2, 4.5) projected
  line L1 (22.2, 4.5) -> (24.3, 4.5)
  line L2 (24.3, -2.46) -> (24.3, 4.5) projected
  line L3 (24.3, 4.5) -> (24.3, -2.46)
  line L4 (24.3, -2.46) -> (39.2, -2.46) projected
  line L5 (24.3, -2.46) -> (39.2, -2.46)
  line L6 (39.2, -2.46) -> (39.2, -29.46) projected
  line L7 (39.2, -2.46) -> (39.2, -29.46)
  line L8 (39.2, -29.46) -> (23.2371, -29.46) projected
  line L9 (39.2, -29.46) -> (23.2371, -29.46)
  line L10 (23.2371, -29.46) -> (23.2371, -34.46) projected
  line L11 (23.2371, -29.46) -> (23.2371, -34.46)
  line L12 (23.2371, -34.46) -> (12.7, -34.46) projected
  line L13 (23.2371, -34.46) -> (12.7, -34.46)
  line L14 (12.7, -25.5) -> (12.7, -24.5) projected
  line L15 (12.7, -34.46) -> (12.7, -24.5)
  line L16 (12.7, -24.5) -> (13.7, -24.5)
  line L17 (13.7, -24.5) -> (13.7, -33.46)
  line L18 (13.7, -33.46) -> (22.2371, -33.46)
  line L19 (22.2371, -33.46) -> (22.2371, -28.46)
  line L20 (22.2371, -28.46) -> (38.2, -28.46)
  line L21 (38.2, -28.46) -> (38.2, -3.46)
  line L22 (38.2, -3.46) -> (23.3, -3.46)
  line L23 (23.3, -3.46) -> (23.3, 3.5)
  line L24 (-7.2, 3.5) -> (22.2, 3.5) projected
  line L25 (22.2, 3.5) -> (23.3, 3.5)
  line L26 (22.2, 3.5) -> (22.2, 4.5) projected
  line L27 (22.2, 3.5) -> (22.2, 4.5)
  line L28 (22.2371, -28.46) -> (22.2371, -27.46)
  line L29 (23.2371, -29.46) -> (39.2, -29.46) projected
  line L30 (23.2371, -29.46) -> (23.2371, -28.46)
  line L31 (22.2371, -27.46) -> (38.2, -27.46)
  line L32 (23.2371, -28.46) -> (38.2, -28.46)
  line L33 (38.2, -28.46) -> (38.2, -29.46)
  line L34 (38.2, -28.46) -> (39.2, -28.46)
  line L35 (23.3, -3.46) -> (23.3, -4.46)
  line L36 (23.3, -4.46) -> (38.2, -4.46)
  line L37 (38.2, -4.46) -> (38.2, -2.46)
  line L38 (24.3, -2.46) -> (24.3, -4.46)
  line L39 (38.2, -3.46) -> (39.2, -3.46)
  line L40 (23.3, -4.46) -> (23.3, -34.46)
  line L41 (23.3, -34.46) -> (24.3, -34.46)
  line L42 (24.3, -34.46) -> (24.3, -3.46)
  line L43 (23.3, -27.46) -> (24.3, -27.46)
  line L44 (22.2371, -33.46) -> (24.3, -33.46)
  line L45 (24.3, -33.46) -> (24.3, -34.46)
  line L46 (22.2371, -34.46) -> (22.2371, -33.46)
  line L47 (22.2371, -34.46) -> (24.3, -34.46)
  point P0 (0, 4.5)
  point P1 (24.3, -3.46)
  point P2 (24.3, -28.46)
  point P3 (23.3, -33.46)
  dimension "d225" = 1
  dimension "d226" = 1
  dimension "d227" = 1
  dimension "d228" = 1
  dimension "d229" = 1
  dimension "d230" = 1
  dimension "d231" = 1
  dimension "d236" = 1
  dimension "d237" = 1
  constraints: 74 end point, 16 point on line, 15 perpendicular, 10 collinear, 5 vertical, 2 horizontal, 1 midpoint, 1 parallel
  measures "d225" distance of L14.end L16.end
  measures "d226" distance between parallel lines of L18 L12
  measures "d227" distance between parallel lines of L10 L19
  measures "d228" distance between parallel lines of L20 L8
  measures "d229" distance between parallel lines of L2 L23
  measures "d230" distance between parallel lines of L4 L22
  measures "d231" distance between parallel lines of L6 L21
  measures "d236" distance of L19.end L28.end
  measures "d237" distance of L22.end L35.end
extrude "Extrusão47" add sketch "Esboço68" along normal blind 12 contours L2 L38 L22 L23 L25 L26 L0 | L38 L36 L35 L22 | L22 L21 L36 L38 | L39 L6 L34 L21 | L42 L20 L40 L31 | L31 L21 L20 L42 | L42 L8 L40 L20 | L42 L44 L40 L8 | L42 L41 L40 L44 | L46 L12 L15 L14 L16 L17 L18 | L44 L10 L12 L46 | L40 L47 L10 L44
fillet "Arredondamento5" radius 2 1 edges at (13.2, 13, 29)
fillet "Arredondamento6" radius 2 1 edges at (22.2, 13, 0.5)
sketch "Esboço69" plane through (0, 1, 4.5) normal (0, 1, 0) x (1, 0, 0)
  line L0 (39.2, -2.46) -> (39.2, -29.46) projected
  line L1 (39.2, -3.46) -> (24.3, -3.46) projected
  line L2 (39.2, -2.46) -> (24.3, -2.46)
  line L3 (24.3, -2.46) -> (24.3, -3.46)
  line L4 (24.3, -3.46) -> (39.2, -3.46)
  line L5 (39.2, -3.46) -> (39.2, -2.46)
  line L6 (39.2, -29.46) -> (23.2371, -29.46) projected
  line L7 (24.3, -28.46) -> (39.2, -28.46) projected
  line L8 (39.2, -29.46) -> (23.2371, -29.46)
  line L9 (23.2371, -29.46) -> (23.2371, -28.46)
  line L10 (23.2371, -28.46) -> (39.2, -28.46)
  line L11 (39.2, -28.46) -> (39.2, -29.46)
  point P0 (0, 4.5)
  constraints: 16 end point, 4 parallel, 2 horizontal, 2 perpendicular
extrude "Extrusão48" cut sketch "Esboço69" against normal blind 12
sketch "Esboço71" plane through (0, 1, 4.5) normal (0, 1, 0) x (1, 0, 0)
  line L0 (23.2371, -28.46) -> (23.2371, -34.46) projected
  line L1 (23.2371, -34.46) -> (24.3, -34.46) projected
  line L2 (23.2371, -34.46) -> (24.3, -34.46)
  line L3 (24.3, -34.46) -> (24.3, -28.46) projected
  line L4 (24.3, -34.46) -> (24.3, -28.46)
  line L5 (39.2, -28.46) -> (23.2371, -28.46) projected
  line L6 (24.3, -28.46) -> (23.2371, -28.46)
  line L7 (23.2371, -28.46) -> (23.2371, -34.46)
  point P0 (0, 4.5)
  constraints: 8 end point, 3 collinear, 1 perpendicular
extrude "Extrusão49" add sketch "Esboço71" against normal blind 1
sketch "Esboço72" plane through (24.3, 0, 32.96) normal (1, 0, 0) x (0, 0, -1)
  line L0 (-6, 0) -> (-6, 13) projected
  line L1 (-6, 0) -> (-3, 0)
  line L2 (0, 0) -> (-6, 0) projected
  line L3 (-3, 0) -> (-3, 13)
  line L4 (1, 13) -> (-5, 13) projected
  line L5 (-3, 13) -> (-3, 6.5)
  circle A0 centre (-3, 6.5) radius 0.5
  line L6 (32.96, 0) -> (2.96, 0) projected
  line L7 (24.9986, 0) -> (30.9986, 0)
  line L8 (30.9986, 0) -> (27.9986, 0)
  line L9 (27.9986, 0) -> (27.9986, 13)
  line L10 (25, 13) -> (32.96, 13) projected
  line L11 (27.9986, 13) -> (27.9986, 6.5)
  circle A1 centre (27.9986, 6.5) radius 0.5
  dimension "d242" = 1
  dimension "d243" = 6
  dimension "d244" = 1
  constraints: 14 end point, 4 midpoint, 4 point on line, 2 centre point, 2 coincident, 2 perpendicular
  measures "d242" diameter of A0
  measures "d243" distance of L7.start L7.end
  measures "d244" diameter of A1
extrude "Extrusão50" cut sketch "Esboço72" against normal blind 1
sketch "Esboço78" plane through (-11.2, -24.2, 0) normal (0, -1, 0) x (1, 0, 0)
  line L0 (0, 30) -> (0, 0) projected
  line L1 (0, 0) -> (14, 0)
  line L2 (0, 0) -> (16.4, 0) projected
  line L3 (14, 0) -> (14, -9.5)
  line L4 (14, -9.5) -> (19.2, -9.5)
  line L5 (19.2, -9.5) -> (19.2, 0)
  line L6 (0, 0) -> (33.4, 0) projected
  line L7 (0, 30) -> (14, 30)
  line L8 (21, 30) -> (11.4, 30) projected
  line L9 (14, 30) -> (14, 39.5)
  line L10 (14, 39.5) -> (19.2, 39.5)
  line L11 (19.2, 39.5) -> (19.2, 30)
  line L12 (17.4, 30) -> (33.4, 30) projected
  line L13 (14, 30) -> (19.2, 30)
  line L14 (19.2, 0) -> (14, 0)
  point P0 (11.2, 0)
  dimension "d247" = 14
  dimension "d248" = 9.5
  dimension "d249" = 5.2
  dimension "d250" = 9.5
  constraints: 20 end point, 6 point on line, 5 perpendicular, 1 horizontal, 1 vertical
  measures "d247" distance of L0.end L1.end
  measures "d248" distance of L1.end L3.end
  measures "d249" distance of L3.end L4.end
  measures "d250" distance of L7.end L9.end
extrude "Extrusão51" add sketch "Esboço78" against normal blind 2
sketch "Esboço79" plane through (-11.2, -24.2, 0) normal (0, -1, 0) x (1, 0, 0)
  line L0 (19.2, -9.5) -> (14, -9.5) projected
  line L1 (14, -9.5) -> (13, -9.5)
  line L2 (13, -9.5) -> (13, 0)
  line L3 (13, 0) -> (13, -9.5)
  line L4 (13, -9.5) -> (13, -10.5)
  line L5 (13, -10.5) -> (19.2, -10.5)
  line L6 (19.2, -10.5) -> (20.2, -10.5)
  line L7 (20.2, -10.5) -> (20.2, 0)
  line L8 (19.2, 0) -> (33.4, 0) projected
  line L9 (20.2, -10.5) -> (20.2, -4.75)
  line L10 (20.2, -4.75) -> (19.2, -4.75)
  line L11 (19.2, 0) -> (19.2, -9.5) projected
  line L12 (19.2, -4.75) -> (19.2, -9.5)
  line L13 (19.2, -9.5) -> (14, -9.5)
  line L14 (13, -10.5) -> (13, -4.75)
  line L15 (13, -10.5) -> (13, -4.75)
  line L16 (13, -4.75) -> (14, -4.75)
  line L17 (14, -9.5) -> (14, 0) projected
  line L18 (14, -4.75) -> (14, -9.5)
  line L19 (13, 0) -> (14, 0)
  line L20 (0, 0) -> (33.4, 0) projected
  line L21 (14, -4.75) -> (14, 0)
  line L22 (0, 30) -> (14, 30) projected
  line L23 (14, 30) -> (13, 30)
  line L24 (13, 30) -> (13, 40.5)
  line L25 (14, 39.5) -> (14, 30) projected
  line L26 (13, 40.5) -> (20.2, 40.5)
  line L27 (19.2, 39.5) -> (14, 39.5) projected
  line L28 (20.2, 40.5) -> (20.2, 30)
  line L29 (19.2, 30) -> (19.2, 39.5) projected
  line L30 (14, 30) -> (14, 39.5)
  line L31 (14, 39.5) -> (19.2, 39.5) projected
  line L32 (14, 39.5) -> (19.2, 39.5)
  line L33 (19.2, 39.5) -> (19.2, 30) projected
  line L34 (19.2, 39.5) -> (19.2, 30)
  line L35 (20.2, 30) -> (19.2, 30)
  line L36 (0, 30) -> (23.9, 30) projected
  line L37 (14, 30) -> (13, 30)
  point P0 (11.2, 0)
  dimension "d253" = 1
  dimension "d254" = 1
  dimension "d255" = 1
  dimension "d256" = 1
  dimension "d257" = 1
  dimension "d258" = 1
  constraints: 52 end point, 11 collinear, 5 point on line, 3 horizontal, 3 perpendicular, 2 midpoint, 2 vertical
  measures "d253" distance of L0.end L1.end
  measures "d254" distance of L1.end L4.end
  measures "d255" distance of L5.end L6.end
  measures "d256" distance between parallel lines of L24 L25
  measures "d257" distance between parallel lines of L26 L27
  measures "d258" distance between parallel lines of L29 L28
extrude "Extrusão52" add sketch "Esboço79" against normal blind 1 contours L11 L10 L7 L6 L5 L4 L1 L0 | L1 L2 L16 L17 | L11 L8 L7 L10 | L16 L2 L19 L17 | L24 L26 L28 L35 L29 L27 L25 L22
sketch "Esboço80" plane through (-11.2, -24.2, 0) normal (0, -1, 0) x (1, 0, 0)
  line L0 (20.2, 0) -> (33.4, 0) projected
  line L1 (20.2, 0) -> (19.2, 0) projected
  line L2 (20.2, 0) -> (19.2, 0)
  line L3 (19.2, -9.5) -> (14, -9.5) projected
  line L4 (19.2, 0) -> (19.2, -9.5)
  line L5 (14, -9.5) -> (14, 0) projected
  line L6 (19.2, -9.5) -> (14, -9.5)
  line L7 (14, -9.5) -> (14, 0)
  line L8 (20.2, -10.5) -> (20.2, 0) projected
  line L9 (20.2, 0) -> (20.2, -10.5)
  line L10 (20.2, -10.5) -> (13, -10.5) projected
  line L11 (20.2, -10.5) -> (13, -10.5)
  line L12 (13, -10.5) -> (13, 0) projected
  line L13 (13, 0) -> (13, -10.5)
  line L14 (13, -10.5) -> (13, -4.75)
  line L15 (13, -4.75) -> (14, -4.75)
  line L16 (19.2, 0) -> (19.2, -9.5) projected
  line L17 (19.2, -4.75) -> (20.2, -4.75)
  line L18 (13, 30) -> (13, 40.5) projected
  line L19 (13, 30) -> (14, 30)
  line L20 (21, 30) -> (11.4, 30) projected
  line L21 (14, 30) -> (14, 39.5) projected
  line L22 (14, 39.5) -> (19.2, 39.5) projected
  line L23 (14, 39.5) -> (19.2, 39.5)
  line L24 (19.2, 39.5) -> (19.2, 30)
  line L25 (19.2, 30) -> (20.2, 30)
  line L26 (20.2, 30) -> (33.4, 30) projected
  line L27 (20.2, 40.5) -> (20.2, 30) projected
  line L28 (20.2, 30) -> (20.2, 40.5)
  line L29 (13, 40.5) -> (20.2, 40.5) projected
  line L30 (20.2, 40.5) -> (13, 40.5)
  line L31 (13, 40.5) -> (13, 30)
  line L32 (14, 39.5) -> (14, 30)
  line L33 (13, 40.5) -> (13, 34.75)
  line L34 (14, 34.75) -> (13, 34.75)
  line L35 (14, 34.75) -> (19.2, 34.75)
  line L36 (19.2, 34.75) -> (20.2, 34.75)
  point P0 (11.2, 0)
  constraints: 44 end point, 11 point on line, 9 perpendicular, 4 collinear, 4 midpoint, 1 vertical
extrude "Extrusão53" add sketch "Esboço80" along normal blind 57 contours L8 L10 L12 L15 L5 L3 L4 L17 | L18 L29 L27 L36 L24 L22 L21 L34
sketch "Esboço81" plane through (-11.2, -23.2, 0) normal (0, 1, 0) x (1, 0, 0)
  line L0 (13, 10.5) -> (13, 0) projected
  line L1 (20.2, 0) -> (20.2, 10.5) projected
  line L2 (13, 10.5) -> (20.2, 10.5)
  line L3 (20.2, 4.75) -> (20.2, 0) projected
  line L4 (20.2, 10.5) -> (20.2, 0)
  line L5 (19.2, 0) -> (19.2, 9.5) projected
  line L6 (19.2, 0) -> (19.2, 9.5)
  line L7 (14, 9.5) -> (14, 0) projected
  line L8 (14, 9.5) -> (14, 0)
  line L9 (0, 0) -> (33.4, 0) projected
  line L10 (14, 0) -> (13, 0)
  line L11 (19.2, 9.5) -> (19.2, 0)
  line L12 (19.2, 9.5) -> (14, 9.5)
  line L13 (19.2, -39.5) -> (19.2, -30) projected
  line L14 (19.2, -30) -> (20.2, -30)
  line L15 (0, -30) -> (23.9, -30) projected
  line L16 (20.2, -40.5) -> (20.2, -30) projected
  line L17 (20.2, -30) -> (20.2, -40.5)
  line L18 (13, -40.5) -> (13, -34.75) projected
  line L19 (20.2, -40.5) -> (13, -40.5) projected
  line L20 (13, -40.5) -> (20.2, -40.5)
  line L21 (20.2, -40.5) -> (13, -40.5)
  line L22 (13, -40.5) -> (13, -30)
  line L23 (13, -30) -> (14, -30)
  line L24 (14, -30) -> (14, -39.5) projected
  line L25 (14, -39.5) -> (19.05, -39.5)
  line L26 (14, -39.5) -> (19.2, -39.5) projected
  line L27 (14, -30) -> (14, -39.5)
  line L28 (19.2, -39.5) -> (19.2, -30)
  line L29 (19.2, -30) -> (20.2, -30)
  line L30 (14, -30) -> (13, -30)
  point P0 (11.2, 0)
  point P1 (14, -30)
  constraints: 36 end point, 8 collinear, 6 point on line, 3 perpendicular, 2 vertical, 1 horizontal, 1 parallel
extrude "Extrusão54" add sketch "Esboço81" along normal blind 1 contours L2 L1 L9 L5 L12 L7 L0 | L13 L14 L16 L19 L18 L22 L15 L24 L25 L26
sketch "Esboço82" plane through (-11.2, -24.2, 0) normal (0, -1, 0) x (1, 0, 0)
  line L0 (16.4, -2) -> (17.4, -2) projected
  line L1 (16.9, -2) -> (16.9, -9.5)
  line L2 (14, -9.5) -> (19.2, -9.5) projected
  line L3 (14, -9.5) -> (16.9, -9.5)
  line L4 (16.9, -9.5) -> (16.9, -2)
  line L5 (16.9, -2) -> (14, -2)
  line L6 (14, -2) -> (14, -9.5)
  line L7 (16.9, -2) -> (19.2, -2)
  line L8 (19.2, -2) -> (19.2, -9.5)
  line L9 (19.2, -9.5) -> (16.9, -9.5)
  line L10 (16.9, -9.5) -> (16.9, -2)
  line L11 (17.4, 32) -> (16.4, 32) projected
  line L12 (16.9, 32) -> (16.9, 39.5)
  line L13 (19.2, 39.5) -> (14, 39.5) projected
  line L14 (14, 39.5) -> (16.9, 39.5)
  line L15 (16.9, 39.5) -> (16.9, 32)
  line L16 (16.9, 32) -> (14, 32)
  line L17 (14, 32) -> (14, 39.5)
  line L18 (19.2, 34.75) -> (19.2, 39.5) projected
  line L19 (16.9, 32) -> (19.2, 32)
  line L20 (19.2, 32) -> (19.2, 39.5)
  line L21 (19.2, 39.5) -> (16.9, 39.5)
  line L22 (16.9, 39.5) -> (16.9, 32)
  point P0 (11.2, 0)
  point P1 (17.4, 32)
  constraints: 36 end point, 8 parallel, 4 horizontal, 4 perpendicular, 2 midpoint, 2 point on line, 2 vertical
extrude "Extrusão55" add sketch "Esboço82" along normal blind 15
sketch "Esboço84" plane through (5, 6.5, 15) normal (1, 0, 0) x (0, 0, -1)
  point P0 (15, -6.5)
